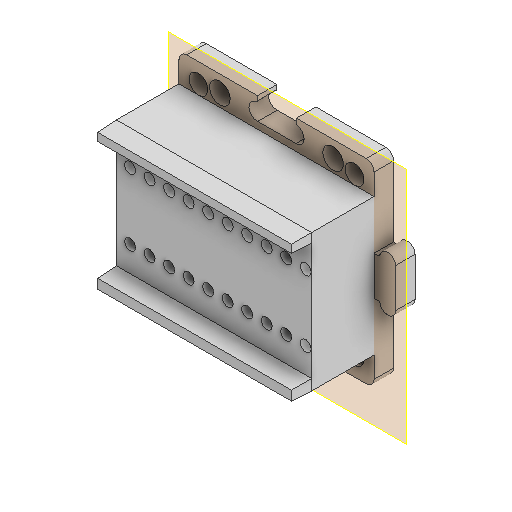
# Autodesk Inventor part: 20_Cube_Insert_Linear_Stage_NEMA11_china_cubemount
Saved by Autodesk Inventor 2022 (Build 260153000, 153)
## iProperties
Created: 2022-01-15
Part Number: 20_Cube_Insert_Linear_Stage_NEMA11_china_cubemount
Material: Generisch
Document SubType Name: Modeling
Designer: diederichbenedict
Density: 1 g/cm^3
Appearance: Vorgabe
Author: diederichbenedict
Autodesk Inventor part; units mm, degrees
ref_plane "YZ Plane" through (0, 0, 0) normal (1, 0, 0) x (0, 1, 0)
ref_plane "XZ Plane" through (0, 0, 0) normal (0, 1, 0) x (-1, 0, 0)
ref_plane "Arbeitsebene1" through (0, 0, 0) normal (0, 0, 1) x (1, 0, 0)
sketch "Skizze1" plane through (0, 0, 0) normal (0, 0, 1) x (1, 0, 0)
  circle A0 centre (5.7948, 15.4052) radius 2.5 projected
  circle A1 centre (-15.6052, -5.7948) radius 2.5 projected
  line L0 (-20.0856, 39.0762) -> (-20.0856, 40.2052) projected
  line L1 (-20.0856, 40.2052) -> (-38.2052, 40.2052) projected
  arc A2 (-38.2052, 40.2052) -> (-40.2052, 38.2052) centre (-38.2052, 38.2052) ccw projected
  line L2 (-40.2052, 20.2953) -> (-40.2052, 38.2052) projected
  line L3 (-40.2052, 20.2953) -> (-39.0783, 20.2953) projected
  arc A3 (-39.0783, 20.2953) -> (-38.6768, 20.6232) centre (-39.0783, 20.7051) ccw projected
  arc A4 (-34.5391, 20.2052) -> (-38.6768, 20.6232) centre (-36.6291, 20.2052) ccw projected
  line L4 (-34.5391, 20.2052) -> (-34.5391, 10.4067) projected
  arc A5 (-38.647, 9.8643) -> (-34.5391, 10.4067) centre (-36.6023, 10.2052) ccw projected
  line L5 (-38.647, 9.8643) -> (-38.6775, 9.9849) projected
  arc A6 (-38.6775, 9.9849) -> (-39.0762, 10.3249) centre (-39.083, 9.9131) ccw projected
  line L6 (-39.0762, 10.3249) -> (-40.2052, 10.3249) projected
  line L7 (-40.2052, -7.7948) -> (-40.2052, 10.3249) projected
  arc A7 (-40.2052, -7.7948) -> (-38.2052, -9.7948) centre (-38.2052, -7.7948) ccw projected
  line L8 (-38.2052, -9.7948) -> (-20.2052, -9.7948) projected
  line L9 (-20.2052, -9.7948) -> (-20.2052, -10.8453) projected
  arc A8 (-20.6052, -11.3352) -> (-20.2052, -10.8453) centre (-20.7052, -10.8453) ccw projected
  arc A9 (-20.6052, -11.3352) -> (-20.2052, -15.2948) centre (-20.2052, -13.2948) ccw projected
  line L10 (-20.2052, -15.2948) -> (-10.2052, -15.2948) projected
  arc A10 (-10.2052, -15.2948) -> (-9.8052, -11.3352) centre (-10.2052, -13.2948) ccw projected
  arc A11 (-10.2052, -10.8453) -> (-9.8052, -11.3352) centre (-9.7052, -10.8453) ccw projected
  line L11 (-10.2052, -10.8453) -> (-10.2052, -9.7948) projected
  line L12 (-10.2052, -9.7948) -> (7.7948, -9.7948) projected
  arc A12 (7.7948, -9.7948) -> (9.7948, -7.7948) centre (7.7948, -7.7948) ccw projected
  line L13 (9.7948, 10.2052) -> (9.7948, -7.7948) projected
  line L14 (9.7948, 10.2052) -> (10.8453, 10.2052) projected
  arc A13 (11.3352, 9.8052) -> (10.8453, 10.2052) centre (10.8453, 9.7052) ccw projected
  arc A14 (11.3352, 9.8052) -> (15.2948, 10.2052) centre (13.2948, 10.2052) ccw projected
  line L15 (15.2948, 10.2052) -> (15.2948, 20.2052) projected
  arc A15 (15.2948, 20.2052) -> (11.3352, 20.6052) centre (13.2948, 20.2052) ccw projected
  arc A16 (10.8453, 20.2052) -> (11.3352, 20.6052) centre (10.8453, 20.7052) ccw projected
  line L16 (10.8453, 20.2052) -> (9.7948, 20.2052) projected
  line L17 (9.7948, 38.2052) -> (9.7948, 20.2052) projected
  arc A17 (9.7948, 38.2052) -> (7.7948, 40.2052) centre (7.7948, 38.2052) ccw projected
  line L18 (7.7948, 40.2052) -> (-10.1151, 40.2052) projected
  line L19 (-10.1151, 40.2052) -> (-10.1151, 39.0783) projected
  arc A18 (-10.1151, 39.0783) -> (-9.7873, 38.6768) centre (-9.7054, 39.0783) ccw projected
  arc A19 (-10.2052, 34.5391) -> (-9.7873, 38.6768) centre (-10.2052, 36.6291) ccw projected
  line L20 (-10.2052, 34.5391) -> (-20.0038, 34.5391) projected
  arc A20 (-20.5462, 38.647) -> (-20.0038, 34.5391) centre (-20.2052, 36.6023) ccw projected
  line L21 (-20.5462, 38.647) -> (-20.4256, 38.6775) projected
  arc A21 (-20.4256, 38.6775) -> (-20.0856, 39.0762) centre (-20.4974, 39.083) ccw projected
  line L22 (-0.2052, 32.2052) -> (-30.2052, 32.2052) projected
  arc A22 (1.7948, 30.2052) -> (-0.2052, 32.2052) centre (-0.2052, 30.2052) ccw projected
  line L23 (1.7948, 30.2052) -> (1.7948, 0.2052) projected
  arc A23 (-0.2052, -1.7948) -> (1.7948, 0.2052) centre (-0.2052, 0.2052) ccw projected
  line L24 (-0.2052, -1.7948) -> (-30.2052, -1.7948) projected
  arc A24 (-32.2052, 0.2052) -> (-30.2052, -1.7948) centre (-30.2052, 0.2052) ccw projected
  line L25 (-32.2052, 0.2052) -> (-32.2052, 30.2052) projected
  arc A25 (-30.2052, 32.2052) -> (-32.2052, 30.2052) centre (-30.2052, 30.2052) ccw projected
  circle A26 centre (-35.2052, 35.2052) radius 2.425 projected
  circle A27 centre (-29.7052, 36.0052) radius 2.65 projected
  circle A28 centre (-36.0052, 29.7052) radius 2.65 projected
  circle A29 centre (-35.2052, -4.7948) radius 2.425 projected
  circle A30 centre (-29.7052, -5.5948) radius 2.65 projected
  circle A31 centre (-36.0052, 0.7052) radius 2.65 projected
  circle A32 centre (4.7948, 35.2052) radius 2.425 projected
  circle A33 centre (-0.7052, 36.0052) radius 2.65 projected
  circle A34 centre (5.5948, 29.7052) radius 2.65 projected
  circle A35 centre (5.5948, 0.7052) radius 2.65 projected
  circle A36 centre (-0.7052, -5.5948) radius 2.65 projected
  circle A37 centre (4.7948, -4.7948) radius 2.425 projected
  point P0 (0, 0)
extrude "Extrusion1" add sketch "Skizze1" against normal blind 5 contours A21 L21 A20 L20 A19 A18 L19 L18 A17 L17 L16 A16 A15 L15 A14 A13 L14 L13 A12 L12 L11 A11 A10 L10 A9 A8 L9 L8 A7 L7 L6 A6 L5 A5 L4 A4 A3 L3 L2 A2 L1 L0 | A22 L23 A23 L24 A24 L25 A25 L22
sketch "Skizze2" plane through (0, 0, 0) normal (0, 0, 1) x (1, 0, 0)
  line L0 (-83.2052, 0.4052) -> (-83.2052, 30.4052) projected
  line L1 (4.7948, 30.4052) -> (-83.2052, 30.4052) projected
  line L2 (4.7948, 0.4052) -> (4.7948, 30.4052) projected
  line L3 (4.7948, 0.4052) -> (-83.2052, 0.4052) projected
  circle A0 centre (-70.2052, 15.4052) radius 1.025 projected
  circle A1 centre (-50.2052, 15.4052) radius 1.025 projected
  circle A2 centre (-30.2052, 15.4052) radius 1.025 projected
  circle A3 centre (-10.2052, 15.4052) radius 1.025 projected
  circle A4 centre (-11.7052, 6.9052) radius 1.7 projected
  circle A5 centre (-11.7052, 23.9052) radius 1.7 projected
  circle A6 centre (-66.7052, 23.9052) radius 1.7 projected
  circle A7 centre (-66.7052, 6.9052) radius 1.7 projected
  circle A8 centre (-15.6052, -5.7948) radius 2.5 projected
  line L4 (-107.8052, 15.4052) -> (29.3948, 15.4052)
  line L5 (-38.2052, -9.7948) -> (-20.2052, -9.7948) projected
  line L6 (-40.2052, 10.3249) -> (-40.2052, -7.7948) projected
  line L7 (9.7948, -7.7948) -> (9.7948, 10.2052) projected
  circle A9 centre (-15.2052, 15.2052) radius 25
  line L8 (9.7948, 20.2052) -> (9.7948, 38.2052) projected
  line L9 (-40.2052, -2.3698) -> (9.7948, -2.3698)
  line L10 (9.7948, -2.3698) -> (9.7948, 32.7802)
  line L11 (9.7948, 32.7802) -> (-40.2052, 32.7802)
  line L12 (-40.2052, 32.7802) -> (-40.2052, -2.3698)
  line L13 (-40.2052, -2.3698) -> (9.7948, 32.7802) construction
  line L14 (9.7948, -2.3698) -> (-40.2052, 32.7802) construction
  circle A10 centre (-35.2052, 35.2052) radius 2.425 projected
  point P0 (0, 0)
  point P1 (9.7948, -2.3698)
  constraints: 14 end point, 4 tangent, 2 horizontal, 2 midpoint, 2 parallel, 1 centre point, 1 perpendicular, 1 point on line, 2 other
ref_plane "Arbeitsebene2" through (4.7948, 0.4052, 16) normal (0, 0, -1) x (0, 1, 0)
extrude "Extrusion2" add sketch "Skizze2" along normal up to surface (16 mm away) contours L6 L12 A9 L3 | L3 A9 L9 L6 | A9 L4 A2 A3 L2 L3 | L3 L2 L4 A9 L9 | L12 L11 A9 L1 | L1 A9 L12 | A9 L1 L2 L4 A3 A2 | A9 L11 L1 | L2 A9 L4 | L4 A2 | A2 L4 | A9 L10 L7 L9 | A9 L11 L8 L10 L2 L1 | L1 L2 A9 | L4 A3 | A3 L4 | A4 | A5
sketch "Skizze3" plane through (-40.2052, -2.3698, 16) normal (0, 0, 1) x (1, 0, 0)
  line L0 (0, 0) -> (50, 0) projected
  line L1 (45, 2.775) -> (-43, 2.775) projected
  line L2 (50, 35.15) -> (0, 35.15) projected
  line L3 (45, 32.775) -> (-43, 32.775) projected
  line L4 (0, 35.15) -> (0, 0) projected
  line L5 (50, 0) -> (0, 0)
  line L6 (0, 0) -> (0, 2.775)
  line L7 (0, 2.775) -> (50, 2.775)
  line L8 (50, 2.775) -> (50, 0)
  line L9 (50, 35.15) -> (0, 35.15)
  line L10 (0, 35.15) -> (0, 32.775)
  line L11 (0, 32.775) -> (50, 32.775)
  line L12 (50, 32.775) -> (50, 35.15)
  point P0 (40.2052, 2.3698)
  point P1 (0, 32.775)
  point P2 (0, 2.775)
  dimension "d4" = 0
  dimension "d5" = 0
  constraints: 16 end point, 4 parallel, 2 horizontal, 2 perpendicular, 2 point on line
  measures "d4" distance between parallel lines of L11 L3
  measures "d5" distance between parallel lines of L1 L7
extrude "Extrusion3" add sketch "Skizze3" along normal blind 5 draft -2
sketch "Skizze4" plane through (-40.2052, 30.4052, 16) normal (0, 0, 1) x (1, 0, 0)
  circle A0 centre (28.5, -23.5) radius 1.7 projected
  circle A1 centre (28.5, -6.5) radius 1.7 projected
  point P0 (40.2052, -30.4052)
hole "Bohrung1" at (-11.7052, 6.9052, 16) at (-11.7052, 23.9052, 16) direction (0, 0, -1) diameter 2.8 end through all
pattern_linear "Rechteckige Anordnung1" count 12 spacing 5 along (1, 0, 0) of "Bohrung1" first direction both ways yes
chamfer "Fase1" distance 0.5 angle 45 15 edges at (-37.6302, 35.2052, -5) (-32.3552, 36.0052, -5) (-38.6552, 29.7052, -5) (-38.6552, 0.7052, -5) (-37.6302, -4.7948, -5) (-32.3552, -5.5948, -5) (-18.1052, -5.7948, -5) (-3.3552, -5.5948, -5) (-3.3552, -5.5948, 0) (2.3698, -4.7948, -5) (2.9448, 0.7052, -5) (3.2948, 15.4052, -5) (2.9448, 29.7052, -5) (2.3698, 35.2052, -5) (-3.3552, 36.0052, -5)
